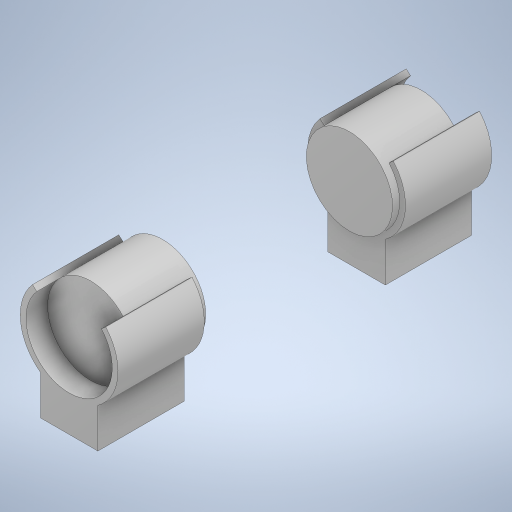
# Autodesk Inventor part: fuse_cover
Saved by Autodesk Inventor 2024.1 (Build 281209000, 209)
## iProperties
Created: 2025-02-19
Part Number: fuse_cover
Material: アルミニウム 6061
Document SubType Name: Modeling
Designer: hibik
Density: 2.7 g/cm^3
Appearance: アルミニウム - フラット
Author: hibik
Autodesk Inventor part; units mm, degrees
ref_plane "YZ Plane" through (0, 0, 0) normal (1, 0, 0) x (0, 1, 0)
ref_plane "XZ Plane" through (0, 0, 0) normal (0, 1, 0) x (-1, 0, 0)
sketch "スケッチ1" plane through (0, 0, 0) normal (0, 1, 0) x (-1, 0, 0)
  line L0 (3.4, 7) -> (-3.4, 7)
  line L1 (-3.4, 7) -> (-3.4, 13)
  line L2 (-3.4, 13) -> (3.4, 13)
  line L3 (3.4, 13) -> (3.4, 7)
  point P0 (0, 0)
  point P1 (0, 7)
  dimension "d0" = 7
  dimension "d1" = 13
  dimension "d2" = 6.8
  constraints: 8 end point, 2 parallel, 1 horizontal, 1 midpoint, 1 perpendicular, 1 vertical alignment
  measures "d0" distance from line of point (0, 0) L0
  measures "d1" distance from line of point (0, 0) L2
  measures "d2" distance of L1.end L2.end
extrude "押し出し1" add sketch "スケッチ1" along normal blind 8.5
sketch "スケッチ2" plane through (-3.4, 0, 13) normal (0, 0, 1) x (1, 0, 0)
  circle A0 centre (3.4, 5.5) radius 3
  line L0 (0, 0) -> (6.8, 0) projected
  line L1 (0, 8.5) -> (6.8, 8.5) projected
  circle A1 centre (3.4, 5.5) radius 3.4
  line L2 (6.8, 0) -> (6.8, 8.5) projected
  line L3 (3.4, 5.5) -> (0, 8.5)
  line L4 (3.4, 5.5) -> (6.8, 8.5)
  line L5 (1.4, 2.7505) -> (5.4, 2.7505)
  line L6 (5.4, 2.7505) -> (5.4, 0)
  line L7 (5.4, 0) -> (1.4, 0)
  line L8 (1.4, 0) -> (1.4, 2.7505)
  line L9 (0, 0) -> (0, 8.5) projected
  point P0 (3.4, 0)
  point P1 (3.4, 0)
  point P2 (3.4, 2.7505)
  point P3 (3.4, 0)
  point P4 (0, 5.5)
  point P5 (0.8506, 7.7495)
  point P6 (1.1505, 7.4849)
  point P7 (5.6495, 7.4849)
  point P8 (5.9494, 7.7495)
  point P9 (6.8, 5.5)
  point P10 (5.4, 2.7505)
  dimension "d5" = 6
  dimension "d6" = 4
  constraints: 12 end point, 3 midpoint, 2 parallel, 2 vertical alignment, 1 centre point, 1 coincident, 1 horizontal, 1 perpendicular, 1 point on line, 1 tangent, 1 vertical, 3 other
  measures "d5" diameter of A0
  measures "d6" distance of L5.start L5.end
extrude "押し出し2" cut sketch "スケッチ2" against normal up to surface (6 mm away) contours A0 L5 L3 L4 | L4 L3 A0 | A0 L1 A1 L4 | A0 L5 | A0 L3 A1 L1 | L4 L2 A1 | A1 L1 L4 | A1 L2 L0 L6 | A1 L3 L1 | L8 L0 L9 A1 | A1 L9 L3
ref_plane "作業平面1" through (-2, 0, 11.5) normal (0, 0, 1) x (1, 0, 0)
sketch "スケッチ5" plane through (-2, 0, 11.5) normal (0, 0, 1) x (1, 0, 0)
  arc A0 (-0.2495, 7.4849) -> (4.2495, 7.4849) centre (2, 5.5) ccw projected
  circle A1 centre (2, 5.5) radius 3
  point P0 (2, 0)
  point P1 (-0.2495, 7.4849)
  constraints: 1 centre point, 1 coincident, 1 concentric
extrude "押し出し5" add sketch "スケッチ5" against normal blind 5
mirror "ミラー1" about plane through (0, 0, 0) normal (0, 0, 1)
